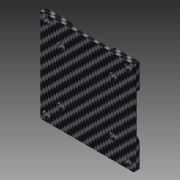
# Autodesk Inventor part: botten
Saved by Autodesk Inventor 2015 (Build 190159000, 159)
## iProperties
Created: 2016-11-27
Part Number: botten
Material: Generic
Document SubType Name: Modeling
Designer: Hampus
Density: 1 g/cm^3
Appearance: Carbon Fiber
Author: Hampus
Autodesk Inventor part; units mm, degrees
ref_plane "YZ Plane" through (0, 0, 0) normal (1, 0, 0) x (0, 1, 0)
ref_plane "XZ Plane" through (0, 0, 0) normal (0, 1, 0) x (-1, 0, 0)
ref_plane "XY Plane" through (0, 0, 0) normal (0, 0, 1) x (1, 0, 0)
sketch "Sketch1" plane through (0, 0, 0) normal (0, 1, 0) x (-1, 0, 0)
  line L0 (0, -32) -> (-32, -32)
  line L1 (-32, -32) -> (-32, 0)
  line L2 (-32, 0) -> (0, 0)
  line L3 (0, 0) -> (0, -32)
  line L4 (0, 0) -> (-4, 0)
  line L5 (-32, 0) -> (-32, -4)
  circle A0 centre (-2, -2) radius 1.25
  circle A1 centre (-30, -2) radius 1.25
  circle A2 centre (-2, -30) radius 1.25
  circle A3 centre (-30, -30) radius 1.25
  line L6 (-8.4853, -32) -> (-14.8492, -25.636)
  line L7 (0, -23.5147) -> (-6.364, -17.1508)
  line L8 (-6.364, -17.1508) -> (-14.8492, -25.636)
  circle A4 centre (-7.0711, -24.9289) radius 1.25
  line L9 (-23.5147, -32) -> (-17.1508, -25.636)
  line L10 (-32, -23.5147) -> (-25.636, -17.1508)
  circle A5 centre (-24.9289, -24.9289) radius 1.25
  line L11 (-25.636, -17.1508) -> (-17.1508, -25.636)
  line L12 (-8.4853, 0) -> (-14.8492, -6.364)
  line L13 (-6.364, -14.8492) -> (-14.8492, -6.364)
  circle A6 centre (-7.0711, -7.0711) radius 1.25
  line L14 (-25.636, -14.8492) -> (-17.1508, -6.364)
  circle A7 centre (-24.9289, -7.0711) radius 1.25
  line L15 (-23.5147, 0) -> (-17.1508, -6.364)
  line L16 (-32, -8.4853) -> (-25.636, -14.8492)
  line L17 (0, -8.4853) -> (-6.364, -14.8492)
  point P0 (0, 0)
  point P1 (0, 0)
  dimension "d0" = 4
  dimension "d1" = 2.5
  dimension "d2" = 2.5
  constraints: 36 end point, 10 point on line, 8 centre point, 2 parallel, 1 perpendicular
  measures "d0" distance of L1.end L5.end
  measures "d1" diameter of A0
  measures "d2" diameter of A1
extrude "Extrusion1" add sketch "Sketch1" along normal blind 1
extrude "Extrusion2" add sketch "Sketch1" along normal blind 2 contours L0 L6 L8 L7 L3 | L0 L1 L10 L11 L9 | L17 L13 L12 L2 L3 | L1 L2 L15 L14 L16
body "Solid1"
